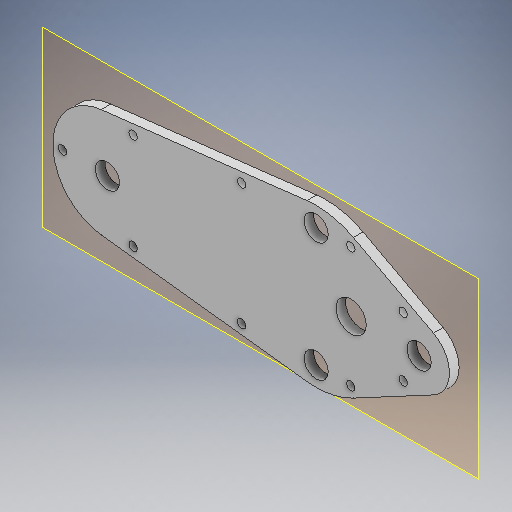
# Autodesk Inventor part: Elo_base
Saved by Autodesk Inventor 2025.2 (Build 292293000, 293)
## iProperties
Created: 2025-04-02
Part Number: Elo_base
Material: Generic
Document SubType Name: Modeling
Designer: Tiago
Density: 1 g/cm^3
Appearance: Default
Author: Tiago
Autodesk Inventor part; units mm, degrees
ref_plane "YZ Plane" through (0, 0, 0) normal (1, 0, 0) x (0, 1, 0)
ref_plane "XZ Plane" through (0, 0, 0) normal (0, 1, 0) x (-1, 0, 0)
sketch "Sketch1" plane through (0, 0, 0) normal (0, 0, 1) x (1, 0, 0)
  line L0 (0, -24.5) -> (0, 24.5) construction
  line L1 (0, 24.5) -> (42.4352, 0) construction
  line L2 (42.4352, 0) -> (0, -24.5) construction
  circle A0 centre (0, 24.5) radius 5
  circle A1 centre (0, -24.5) radius 5
  circle A2 centre (42.4352, 0) radius 5
  line L3 (48.3266, 11.0246) -> (15.3175, 28.664)
  line L4 (48.3266, -11.0246) -> (15.3175, -28.664)
  arc A3 (31.6099, -6.25) -> (31.822, -6.6037) centre (42.4352, 0) ccw
  arc A4 (31.822, -6.6037) -> (31.9289, -6.0658) centre (0, 0) ccw
  arc A5 (31.9289, 6.0658) -> (31.822, 6.6037) centre (0, 0) ccw
  arc A6 (48.3266, -11.0246) -> (48.3266, 11.0246) centre (42.4352, 0) ccw
  arc A7 (31.822, 6.6037) -> (31.6099, 6.25) centre (42.4352, 0) ccw
  line L5 (42.4352, 0) -> (14.4352, 0) construction
  circle A8 centre (14.4352, 0) radius 6.25
  line L6 (0, 0) -> (-86, 0) construction
  arc A9 (-88.6163, 22.3474) -> (-88.6163, -22.3474) centre (-86, 0) ccw
  line L7 (-88.6163, 22.3474) -> (-3.7791, 32.2795)
  line L8 (-88.6163, -22.3474) -> (-3.7791, -32.2795)
  arc A10 (15.3175, 28.664) -> (-3.7791, 32.2795) centre (0, 0) ccw
  arc A11 (-3.7791, -32.2795) -> (15.3175, -28.664) centre (0, 0) ccw
  circle A12 centre (-86, 0) radius 5
  line L9 (-86, 0) -> (-104.5, 0) construction
  circle A13 centre (-104.5, 0) radius 1.75
  line L10 (-86, 0) -> (-75.3956, 19.8443) construction
  circle A14 centre (-75.3956, 19.8443) radius 1.75
  line L11 (-75.3956, 19.8443) -> (-30.7009, 25.0769) construction
  line L12 (-31.1687, 29.0729) -> (-30.7036, 25.1001) construction
  circle A15 centre (-30.7036, 25.1001) radius 1.75
  line L13 (-30.7036, 25.1001) -> (14.2964, 25.1001) construction
  line L14 (15.3175, 28.664) -> (14.2964, 24.7965) construction
  circle A16 centre (14.2964, 24.7965) radius 1.75
  line L15 (14.2964, 24.7965) -> (35.904, 12.2222) construction
  circle A17 centre (35.904, 12.2222) radius 1.75
  circle A18 centre (-75.3956, -19.8443) radius 1.75
  circle A19 centre (-30.7036, -25.1001) radius 1.75
  circle A20 centre (14.2964, -24.7965) radius 1.75
  circle A21 centre (35.904, -12.2222) radius 1.75
  dimension "d1" = 49
  dimension "d2" = 49
  dimension "d3" = 10
  dimension "d4" = 10
  dimension "d5" = 10
  dimension "d7" = 28
  dimension "d8" = 12.5
  dimension "d9" = 86
  dimension "d10" = 45
  dimension "d11" = 10
  dimension "d12" = 18.5
  dimension "d13" = 3.5
  dimension "d14" = 3.5
  dimension "d15" = 45
  dimension "d16" = 4
  dimension "M4" = 3.5
  dimension "d18" = 45
  dimension "d19" = 4
  dimension "d20" = 3.5
  dimension "d22" = 25
  dimension "d26" = 3.5
  constraints: 32 end point, 22 centre point, 16 point on circle, 13 coincident, 8 tangent, 5 point on line, 4 horizontal, 4 symmetric about line, 1 horizontal alignment, 1 midpoint, 1 vertical, 4 other
  measures "d1" distance of L0.start L0.end
  measures "d2" distance of L0.end L1.end
  measures "d3" diameter of A0
  measures "d4" diameter of A1
  measures "d5" diameter of A2
  measures "d7" distance of L5.start L5.end
  measures "d8" diameter of A8
  measures "d9" distance of L6.start L6.end
  measures "d10" diameter of A9
  measures "d11" diameter of A12
  measures "d12" distance of L9.start L9.end
  measures "d13" diameter of A13
  measures "d14" diameter of A14
  measures "d15" distance of L11.start L11.end
  measures "d16" distance of L12.start L12.end
  measures "M4" diameter of A15
  measures "d18" distance of L13.start L13.end
  measures "d19" distance of L3.end L14.end
  measures "d20" diameter of A16
  measures "d22" distance of L15.start L15.end
  measures "d26" diameter of A17
extrude "Extrusion1" add sketch "Sketch1" along normal blind 4
equation "\"d13\" = M4"
equation "\"d14\" = M4"
equation "\"d20\" = M4"
equation "\"d26\" = M4"
body "Solid1"
